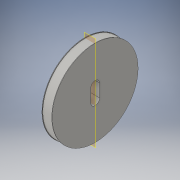
# Autodesk Inventor part: msheehan_wheel
Saved by Autodesk Inventor 2016 (Build 200138000, 138)
## iProperties
Created: 2017-08-31
Part Number: msheehan_wheel
Material: Generic
Document SubType Name: Modeling
Designer: student
Density: 1 g/cm^3
Appearance: Default
Author: student
Autodesk Inventor part; units mm, degrees
ref_plane "YZ Plane" through (0, 0, 0) normal (1, 0, 0) x (0, 1, 0)
ref_plane "XZ Plane" through (0, 0, 0) normal (0, 1, 0) x (-1, 0, 0)
sketch "Sketch1" plane through (0, 0, 0) normal (1, 0, 0) x (0, 1, 0)
  circle A0 centre (0, 0) radius 23.114
  dimension "d0" = 46.228
  constraints: 1 centre point, 1 coincident
  measures "d0" diameter of A0
extrude "Extrusion1" add sketch "Sketch1" along normal blind 5.588
sketch "Sketch3" plane through (0, 0, 0) normal (0, 0, 1) x (1, 0, 0)
  line L0 (5.588, -23.114) -> (5.588, 23.114) projected
  line L1 (5.588, 23.114) -> (5.588, 23.368)
  line L2 (5.588, 23.368) -> (5.334, 23.368)
  line L3 (5.334, 23.368) -> (5.334, 23.114)
  line L4 (0, 23.114) -> (5.588, 23.114) projected
  line L5 (5.334, 23.114) -> (5.588, 23.114)
  line L6 (0, 0) -> (5.588, 0)
  line L7 (0, 23.114) -> (0, 23.368)
  line L8 (0, 23.368) -> (0.254, 23.368)
  line L9 (0.254, 23.368) -> (0.254, 23.114)
  line L10 (0, 23.114) -> (0.254, 23.114)
  dimension "d5" = 0.254
  dimension "d6" = 0.254
  dimension "d7" = 0.254
  dimension "d8" = 0.254
  constraints: 18 end point, 4 perpendicular, 2 collinear, 2 point on line, 2 vertical, 1 midpoint
  measures "d5" distance of L0.end L1.end
  measures "d6" distance of L1.end L2.end
  measures "d7" distance of L4.start L7.end
  measures "d8" distance of L7.end L8.end
revolve "Revolution1" add sketch "Sketch3" angle 360 about axis through (0, 0, 0) along (1, 0, 0)
sketch "Sketch4" plane through (5.588, 0, 0) normal (1, 0, 0) x (0, 0, -1)
  line L0 (0, -3.4925) -> (0, 3.4925) construction
  line L1 (2.413, -3.4925) -> (2.413, 3.4925)
  line L2 (-2.413, 3.4925) -> (-2.413, -3.4925)
  arc A0 (-2.413, -3.4925) -> (2.413, -3.4925) centre (0, -3.4925) ccw
  arc A1 (2.413, 3.4925) -> (-2.413, 3.4925) centre (0, 3.4925) ccw
  point P0 (0, 0)
  dimension "d10" = 3.4925
  dimension "d11" = 4.826
  constraints: 8 end point, 4 point on circle, 4 tangent, 2 centre point, 1 midpoint, 1 parallel, 1 vertical
  measures "d10" distance of point (0, 0) L0.end
  measures "d11" diameter of A1
extrude "Extrusion2" cut sketch "Sketch4" against normal blind 5.08
body "Solid1"
